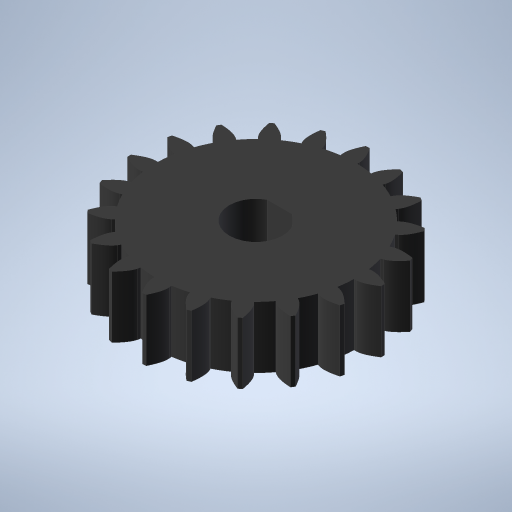
# Autodesk Inventor part: inner arm pinion
Saved by Autodesk Inventor 2024 (Build 280153000, 153)
## iProperties
Created: 2024-04-06
Part Number: inner arm pinion
Material: Generic
Document SubType Name: Modeling
Designer: drew
Density: 1 g/cm^3
Appearance: Default
Author: drew
Autodesk Inventor part; units mm, degrees
ref_plane "YZ Plane" through (0, 0, 0) normal (1, 0, 0) x (0, 1, 0)
ref_plane "XZ Plane" through (0, 0, 0) normal (0, 1, 0) x (-1, 0, 0)
ref_plane "XY Plane" through (0, 0, 0) normal (0, 0, 1) x (1, 0, 0)
sketch "Sketch1" plane through (0, 0, 0) normal (0, 1, 0) x (-1, 0, 0)
  circle A0 centre (0, 0) radius 10.5833 construction
  line L0 (8.4413, 5.8851) -> (13.2655, -7.3691) construction
  line L1 (0, 0) -> (10.5833, 0) construction
  line L2 (10.5833, 0) -> (10.5833, -9.372)
  circle A1 centre (0, 0) radius 9.9451 construction
  line L3 (0, 0) -> (9.3453, 3.4014) construction
  arc A2 (9.3453, 3.4014) -> (7.9128, 6.0243) centre (0, 0) ccw
  line L4 (7.9128, 6.0243) -> (0, 0) construction
  line L5 (7.9128, 6.0243) -> (11.9227, 0.7574) construction
  arc A3 (9.7503, 1.9586) -> (9.3453, 3.4014) centre (0, 0) ccw
  line L6 (9.7503, 1.9586) -> (10.1678, -0.1196) construction
  arc A4 (9.944, -0.1482) -> (9.3453, 3.4014) centre (0, 0) ccw
  dimension "d0" = 21.1667
  dimension "d1" = 20
  dimension "d2" = 3.6197
  dimension "d3" = 3
  dimension "d4" = 6.6197
  dimension "d6" = 1.5
  dimension "d7" = 2.1197
  dimension "d8" = 3.6197
  constraints: 14 end point, 6 point on circle, 5 coincident, 5 point on line, 3 centre point, 2 tangent, 1 horizontal, 1 horizontal alignment, 1 vertical, 11 other
  measures "d1" angle of L2 L0
  measures "d2" distance of L1.end L3.end
  measures "d4" distance of L4.start L5.end
  measures "d7" distance of L6.start L6.end
sketch "Sketch2" plane through (0, 0, 0) normal (0, 1, 0) x (-1, 0, 0)
  spline S0 degree 3 poles (11.9227, 0.7574) (10.7634, -0.0402) (10.2802, -0.1197) (9.944, -0.1482) knots 0 0 0 0 1 1 1 1
  line L0 (0, 0) -> (9.944, -0.1482) construction
  line L1 (0, 0) -> (9.8915, 0.6303) construction
  spline S1 degree 3 poles (11.9224, 0.7621) (10.6712, 1.406) (10.1818, 1.4235) (9.8447, 1.4092) knots 0 0 0 0 1 1 1 1
  circle A0 centre (0, 0) radius 11.6417 construction
  line L2 (9.944, -0.1482) -> (9.694, -0.1445)
  line L3 (9.8447, 1.4092) -> (9.5973, 1.3738)
  circle A1 centre (0, 0) radius 9.6951 construction
  point P0 (10.5833, 0)
  point P1 (10.1678, -0.1196)
  point P2 (10.4977, 1.3433)
  point P3 (10.0704, 1.4092)
  dimension "d9" = 4.5
  dimension "d10" = 23.2833
  dimension "d11" = 0.25
  constraints: 8 end point, 5 symmetric about line, 2 coincident, 1 centre point, 1 point on line, 11 other
  measures "d9" angle of L1 L0
  measures "d10" diameter of A0
  measures "d11" distance of L0.end L2.end
sketch "Sketch3" plane through (0, 0, 0) normal (0, 1, 0) x (-1, 0, 0)
  circle A0 centre (0, 0) radius 9.6951 construction
  spline S0 degree 3 poles (11.9227, 0.7574) (10.7634, -0.0402) (10.2802, -0.1197) (9.944, -0.1482) knots 0 0 0 0 1 1 1 1 projected
  spline S1 degree 3 poles (11.9224, 0.7621) (10.6712, 1.406) (10.1818, 1.4235) (9.8447, 1.4092) knots 0 0 0 0 1 1 1 1 projected
  line L0 (9.8447, 1.4092) -> (9.5973, 1.3738) projected
  line L1 (0, 0) -> (9.944, -0.1482) construction
  circle A1 centre (0, 0) radius 11.6417 construction
  circle A2 centre (0, 0) radius 9.6951
  constraints: 1 centre point, 1 coincident, 2 other
extrude "Extrusion1" add sketch "Sketch3" along normal mid plane 6
sketch "Sketch4" plane through (0, 0, 0) normal (0, 1, 0) x (-1, 0, 0)
  line L0 (9.8447, 1.4092) -> (9.5973, 1.3738) projected
  spline S0 degree 3 poles (11.9224, 0.7621) (10.6712, 1.406) (10.1818, 1.4235) (9.8447, 1.4092) knots 0 0 0 0 1 1 1 1 projected
  spline S1 degree 3 poles (11.9227, 0.7574) (10.7634, -0.0402) (10.2802, -0.1197) (9.944, -0.1482) knots 0 0 0 0 1 1 1 1 projected
  line L1 (0, 0) -> (9.944, -0.1482) construction
  line L2 (9.944, -0.1482) -> (9.6428, -0.1437)
  line L3 (9.6428, -0.1437) -> (9.5973, 1.3738)
  circle A0 centre (0, 0) radius 11.6417 construction
  arc A1 (11.6282, 0.5606) -> (11.6053, 0.9199) centre (0, 0) ccw
  constraints: 4 end point, 4 point on circle, 1 centre point, 1 coincident, 1 point on line, 2 other
extrude "Extrusion2" add sketch "Sketch4" along normal mid plane 6
pattern_circular "Circular Pattern1" count 20 over 360 about axis through (0, -10, 0) along (0, 1, 0) of "Extrusion2"
sketch "Sketch5" plane through (0, 3, 0) normal (0, 1, 0) x (1, 0, 0)
  arc A0 (-1.2124, 2.3) -> (1.2124, 2.3) centre (0, 0) ccw
  line L0 (-1.2124, 2.3) -> (1.2124, 2.3)
  dimension "d19" = 5.2
  dimension "d20" = 2.3
  constraints: 2 end point, 2 point on circle, 1 centre point, 1 coincident, 1 horizontal
  measures "d19" diameter of A0
  measures "d20" distance from line of point (0, 0) L0
extrude "Extrusion3" cut sketch "Sketch5" against normal through all
equation "\"d0\" = dia"
equation "\"d4\" = d3 + d2"
equation "\"d7\" = d2 - d6"
equation "\"d8\" = d2"
equation "\"d10\" = dia + 2 * mod"
equation "\"dia\" = 21.16667"
equation "\"mod\" = 1.05833"
body "Solid1"
